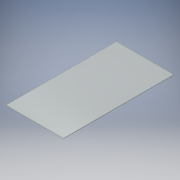
# Autodesk Inventor part: Glass
Saved by Autodesk Inventor 2016 (Build 200138000, 138)
## iProperties
Created: 2016-02-09
Part Number: Glass
Material: Glass
Document SubType Name: Modeling
Designer: ron
Density: 2.18 g/cm^3
Appearance: Clear
Mass: 11610.2 g
Surface Area: 17019.3 cm^2
Volume: 5325.8 cm^3
Author: ron
Autodesk Inventor part; units mm, degrees
ref_plane "YZ Plane" through (0, 0, 0) normal (1, 0, 0) x (0, 1, 0)
ref_plane "XZ Plane" through (0, 0, 0) normal (0, 1, 0) x (-1, 0, 0)
ref_plane "XY Plane" through (0, 0, 0) normal (0, 0, 1) x (1, 0, 0)
sketch "Sketch1" plane through (0, 0, 0) normal (0, 1, 0) x (-1, 0, 0)
  line L0 (0, 0) -> (660.4, 0)
  line L1 (660.4, 0) -> (660.4, -1270)
  line L2 (660.4, -1270) -> (0, -1270)
  line L3 (0, -1270) -> (0, 0)
  dimension "d0" = 660.4
  dimension "d1" = 1270
  constraints: 8 end point, 2 parallel, 1 horizontal, 1 perpendicular
  measures "d0" distance of L1.end L2.end
  measures "d1" distance of L0.end L1.end
extrude "Extrusion1" add sketch "Sketch1" along normal blind 6.35
body "Solid1"
